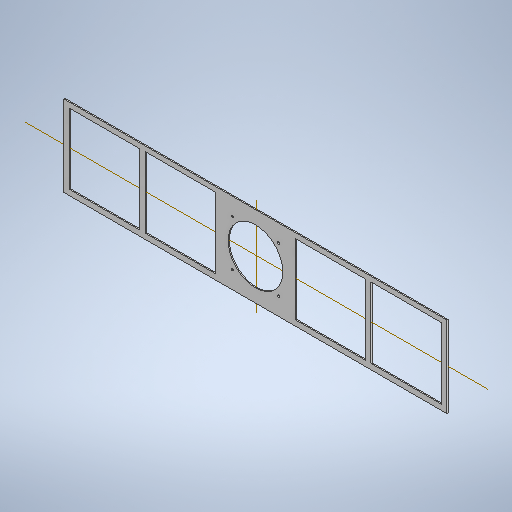
# Autodesk Inventor part: 가로로만
Saved by Autodesk Inventor 2025.1 (Build 291241000, 241)
## iProperties
Created: 2024-10-29
Part Number: 가로로만
Material: 일반
Document SubType Name: Modeling
Designer: gmsee
Density: 1 g/cm^3
Appearance: 기본값
Author: gmsee
Autodesk Inventor part; units mm, degrees
ref_plane "YZ Plane" through (0, 0, 0) normal (1, 0, 0) x (0, 1, 0)
ref_plane "XZ Plane" through (0, 0, 0) normal (0, 1, 0) x (-1, 0, 0)
ref_plane "XY Plane" through (0, 0, 0) normal (0, 0, 1) x (1, 0, 0)
sketch "스케치1" plane through (0, 0, 0) normal (0, 0, 1) x (1, 0, 0)
  line L0 (-350, 74) -> (350, 74)
  line L1 (350, 74) -> (350, -74)
  line L2 (350, -74) -> (-350, -74)
  line L3 (-350, -74) -> (-350, 74)
  line L4 (-340, 64.5) -> (-211.5, 64.5)
  line L5 (-211.5, 64.5) -> (-211.5, -64)
  line L6 (-211.5, -64) -> (-340, -64)
  line L7 (-340, -64) -> (-340, 64.5)
  line L8 (-201.5, 65) -> (-72.5, 65)
  line L9 (-72.5, 65) -> (-72.5, -64)
  line L10 (-72.5, -64) -> (-201.5, -64)
  line L11 (-201.5, -64) -> (-201.5, 65)
  line L12 (211, 65) -> (340, 65)
  line L13 (340, 65) -> (340, -64)
  line L14 (340, -64) -> (211, -64)
  line L15 (211, -64) -> (211, 65)
  line L16 (72.5, 64.5) -> (201, 64.5)
  line L17 (201, 64.5) -> (201, -64)
  line L18 (201, -64) -> (72.5, -64)
  line L19 (72.5, -64) -> (72.5, 64.5)
  circle A0 centre (0, 0) radius 50
  circle A1 centre (42.072, 42.072) radius 2
  circle A2 centre (-42.072, 42.072) radius 2
  circle A3 centre (-42.072, -42.072) radius 2
  circle A4 centre (42.072, -42.072) radius 2
  line L20 (-490, 0) -> (490, 0) projected
  line L21 (0, -103.6) -> (0, 103.6) projected
  point P0 (0, -74)
  point P1 (-72.5, 0.5)
  point P2 (-201.5, 0.5)
  point P3 (-137, -64)
  point P4 (-137, 65)
  point P5 (340, 0.5)
  point P6 (211, 0.5)
  point P7 (275.5, -64)
  point P8 (275.5, 65)
  point P9 (136.75, -64)
  point P10 (136.75, 64.5)
  point P11 (201, 0.25)
  point P12 (72.5, 0.25)
  dimension "d0" = 148
  dimension "d1" = 74
  dimension "d2" = 700
  dimension "d3" = 350
  dimension "d4" = 128.5
  dimension "d5" = 128.5
  dimension "d6" = 10
  dimension "d7" = 10
  dimension "d8" = 129
  dimension "d9" = 129
  dimension "d10" = 10
  dimension "d11" = 10
  dimension "d12" = 129
  dimension "d13" = 129
  dimension "d14" = 128.5
  dimension "d15" = 128.5
  dimension "d16" = 10
  dimension "d17" = 10
  dimension "d18" = 10
  dimension "d19" = 10
  dimension "d20" = 100
  dimension "d21" = 4
  dimension "d22" = 4
  dimension "d23" = 4
  dimension "d24" = 4
  dimension "d25" = 42.072
  dimension "d26" = 42.072
  dimension "d27" = 42.072
  dimension "d28" = 42.072
  dimension "d29" = 42.072
  dimension "d30" = 42.072
  dimension "d31" = 42.072
  dimension "d32" = 42.072
  constraints: 40 end point, 13 midpoint, 10 parallel, 5 centre point, 5 horizontal, 5 perpendicular, 1 coincident
  measures "d0" distance between parallel lines of L2 L0
  measures "d1" distance of point (0, -74) point (0, 0)
  measures "d2" distance between parallel lines of L1 L3
  measures "d3" distance from line of L3 point (0, 0)
  measures "d4" distance between parallel lines of L6 L4
  measures "d5" distance between parallel lines of L5 L7
  measures "d6" distance between parallel lines of L3 L7
  measures "d7" distance between parallel lines of L2 L6
  measures "d8" distance of point (-72.5, 0.5) point (-201.5, 0.5)
  measures "d9" distance of point (-137, -64) point (-137, 65)
  measures "d10" distance between parallel lines of L2 L10
  measures "d11" distance between parallel lines of L11 L5
  measures "d12" distance of point (340, 0.5) point (211, 0.5)
  measures "d13" distance of point (275.5, -64) point (275.5, 65)
  measures "d14" distance of point (136.75, -64) point (136.75, 64.5)
  measures "d15" distance of point (201, 0.25) point (72.5, 0.25)
  measures "d16" distance between parallel lines of L1 L13
  measures "d17" distance between parallel lines of L2 L14
  measures "d18" distance between parallel lines of L18 L2
  measures "d19" distance between parallel lines of L15 L17
  measures "d20" diameter of A0
  measures "d21" diameter of A1
  measures "d22" diameter of A2
  measures "d23" diameter of A4
  measures "d24" diameter of A3
  measures "d25" distance from line of L20 A1.centre
  measures "d26" distance from line of L21 A1.centre
  measures "d27" distance from line of L21 A2.centre
  measures "d28" distance from line of L20 A2.centre
  measures "d29" distance from line of L21 A3.centre
  measures "d30" distance from line of L20 A3.centre
  measures "d31" distance from line of L20 A4.centre
  measures "d32" distance from line of L21 A4.centre
extrude "돌출3" add sketch "스케치1" along normal blind 2 contours L0 L21 A0 L20 L9 L8 L11 L5 L4 L7 L3 | L0 L1 L20 L13 L12 L15 L17 L16 L19 A0 L21 | L20 L7 L6 L5 L11 L10 L9 A0 L21 L2 L3 | L1 L2 L21 A0 L20 L19 L18 L17 L15 L14 L13
equation "\"d1\" = 0.5 * d0"
equation "\"d3\" = 0.5 * d2"
